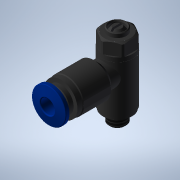
# Autodesk Inventor part: 193138 GRLA-M5-QS-4-D
Saved by Autodesk Inventor 2021 (Build 250183000, 183)
## iProperties
Created: 2026-04-07
Part Number: 193138 GRLA-M5-QS-4-D
Material: Generic
Catalog Web Link: www.3dfindit.com
Description: GRLA-D-one-way flow control valve
Vendor: FESTO
Document SubType Name: Modeling
Designer: psAdmin
Manufacturer: FESTO
Mass: 13 g
Surface Area: 17.273 cm^2
Volume: 2.07274 cm^3
Density: 1 g/cm^3
Appearance: PSOLRGB-176-176-176
Category: PARTsolutions
Company: FESTO
Title: 193138 GRLA-M5-QS-4-D
Author: Cadenas PARTsolutions
Comments: one-way flow control valve
PSOL_IDENT_0: {$CADENAS_DATA/23d-libs/festo/parts/g/grla/grla_d.prj},182 {VTYP=3D},{NB=193138 GRLA-M5-QS-4-D},{LIN
PSOL_IDENT_1: A=193138 GRLA-M5-QS-4-D},{NN=GRLA-D},{DATE=02.05.2025 09:35:38},{GEOMDATE=20.03.2025 09:32:41},{VERS
PSOL_IDENT_2: ION=},{LINEID=20},{WBVAR=},{WBNUMERIC=}  {NB=193138 GRLA-M5-QS-4-D},{LINA=193138 GRLA-M5-QS-4-D},{KT=
PSOL_IDENT_3: DUMMY},{TNR=193138},{TYP=GRLA-M5-QS-4-D},{INFO=},{FDTQS=46},{FDTQSV2=46},{FDTQS1=34},{FDTQS2=346},{F
PSOL_IDENT_4: DTQSDGST=-},{ZOLL=5},{VERS=1.000},{D=M5},{QS=QS-4},{ESTE=-},{DFC=-},{B=9.800},{DP=5.000},{KDRD=4.018
PSOL_IDENT_5: },{D1=8.900},{D2=10.000},{DS=4.000},{H=24.700},{H1=20.300},{L=20.800},{L1=3.350},{L2=10.700},{SW=8.0
PSOL_IDENT_6: 00},{CNSMASSEXACT=0.01300},{MOM=0.8 ±0.1},{GB=0.500},{LHT=1.200},{TW=0.700},{DW=8.400},{DHT=5.200},{
PSOL_IDENT_7: DCH=7.500},{DH=8.900},{HH=4.750},{HHB=5.950},{DI=2.000},{DIH=4.200},{LIH=0.400},{LTS=1.200},{DSJ1=7.
PSOL_IDENT_8: 200},{DSJ2=0.000},{TSJ=0.000},{LSJ1=5.450},{LSJ2=16.400},{ASJ=45.000},{LSJ3=1.815},{LSJ4=9.800},{LSJ
PSOL_IDENT_9: 5=3.300},{LSJ6=0.200},{DSJ3=4.200},{DSJ4=9.900},{DQS=0.000},{LQS=0.000},{DSJ5=7.500},{RSJ1=0.200},{R
PSOL_IDENT_10: SJ2=0.300},{DSJ6=5.400},{DSR=7.800},{TSR=0.500},{DSJ7=9.700},{HN=0.000},{DN=0.000},{DIN=0.000},{DNC=
PSOL_IDENT_11: 0.000},{CHN=0.000},{RN=0.000},{HKH=0.000},{DKH=0.000},{DIKH=0.000},{DKHC=0.000},{CHKH=0.000},{CHKH1=
PSOL_IDENT_12: 0.000},{RKH=0.000},{TKHS=0.000},{HSJ=0.000},{HSJN=0.000},{DAS=0.000},{TIH=1.520},{SRGH=0.150},{DISR=
PSOL_IDENT_13: 7.300},{TQS=15.000},{EOLDATE=},{GTIN=4052568043803},{REACH=Ja},{REACHSVHC=Nein},{REACHHAZSUBS=-},{RE
PSOL_IDENT_14: ACHSCIP=-},{REACHVALDATE=-}
NB: 193138 GRLA-M5-QS-4-D
NN: GRLA-D
NT: one-way flow control valve
NBSYN: $TNR. $TYP.
LINA: 193138 GRLA-M5-QS-4-D
CATALOG: Festo
TNR: 193138
TYP: GRLA-M5-QS-4-D
D: M5
QS: QS-4
ESTE: -
DFC: -
B: 9.8
D1: 8.9
D2: 10
DS: 4
H: 24.7
H1: 20.3
L: 20.8
L1: 3.35
L2: 10.7
SW: 8
CNSMASSEXACT: 0.013
MOM: 0.8 ±0.1
GTIN: 4052568043803
REACH: Yes
REACHSVHC: No
REACHHAZSUBS: -
REACHSCIP: -
REACHVALDATE: -
SUPPLIER: FESTO
ARTICLENO: 193138 GRLA-M5-QS-4-D
BOMINFO: 193138 GRLA-M5-QS-4-D
CREATOR: CADENAS GmbH
Autodesk Inventor part; units mm, degrees
sketch "Sketch_6" plane through (0, 0, 0) normal (0, 0, 1) x (1, 0, 0)
  line L0 (0, -14.05) -> (0, 10.1)
  line L1 (0, 10.1) -> (1.2, 10.1)
  line L2 (1.2, 10.1) -> (2.1, 8.9)
  line L3 (2.1, 8.9) -> (2.1, 9.7)
  line L4 (2.1, 9.7) -> (2.2865, 10.1)
  line L5 (2.2865, 10.1) -> (2.4, 10.1)
  line L6 (2.4, 10.1) -> (2.6, 9.9)
  line L7 (2.6, 9.9) -> (2.6, 8.9)
  line L8 (2.6, 8.9) -> (3.75, 8.9)
  line L9 (3.75, 8.9) -> (4.45, 8.4959)
  line L10 (4.45, 8.4959) -> (4.45, 4.15)
  line L11 (4.45, 4.15) -> (3.75, 4.15)
  line L12 (3.75, 4.15) -> (3.75, 4.1)
  line L13 (3.75, 4.1) -> (4.45, 4.1)
  line L14 (4.45, 4.1) -> (4.45, -9.65)
  line L15 (4.45, -9.65) -> (3.7264, -9.65)
  arc A0 (3.7264, -9.65) -> (3.95, -9.75) centre (3.95, -9.45) ccw
  line L16 (3.95, -9.75) -> (4.2, -9.75)
  line L17 (4.2, -9.75) -> (4.2, -10.45)
  line L18 (4.2, -10.45) -> (3.9, -10.45)
  line L19 (3.9, -10.45) -> (3.9, -10.7)
  line L20 (3.9, -10.7) -> (2.5, -10.7)
  line L21 (2.5, -10.7) -> (2.5, -13.5595)
  line L22 (2.5, -13.5595) -> (2.0095, -14.05)
  line L23 (2.0095, -14.05) -> (0, -14.05)
  line L24 (0, -14.05) -> (0, 10.1)
  constraints: 50 end point, 2 point on circle, 1 centre point
revolve "Revolution1" add sketch "Sketch_6" angle 360 about axis through (0, -14.05, 0) along (0, -1, 0)
thread "Thread1" size "M5x0.8" class "6g" standard "ISO Metric profile" full length
sketch "Sketch_8" plane through (0, 10.1, 0) normal (0, 1, 0) x (1, 0, 0)
  line L0 (-0.3, 1.9774) -> (-0.3, -1.9774)
  arc A0 (-0.3, -1.9774) -> (0.3, -1.9774) centre (0, 0) ccw
  line L1 (0.3, -1.9774) -> (0.3, 1.9774)
  arc A1 (0.3, 1.9774) -> (-0.3, 1.9774) centre (0, 0) ccw
  constraints: 4 end point, 4 point on circle, 2 centre point
extrude "Extrusion1" cut sketch "Sketch_8" against normal blind 1
sketch "Sketch_15" plane through (0, 10.1, 0) normal (0, 1, 0) x (1, 0, 0)
  line L0 (-8, -4.6188) -> (0, -9.2376)
  line L1 (0, -9.2376) -> (8, -4.6188)
  line L2 (8, -4.6188) -> (8, 4.6188)
  line L3 (8, 4.6188) -> (0, 9.2376)
  line L4 (0, 9.2376) -> (-8, 4.6188)
  line L5 (-8, 4.6188) -> (-8, -4.6188)
  line L6 (-4, -2.3094) -> (0, -4.6188)
  line L7 (0, -4.6188) -> (4, -2.3094)
  line L8 (4, -2.3094) -> (4, 2.3094)
  line L9 (4, 2.3094) -> (0, 4.6188)
  line L10 (0, 4.6188) -> (-4, 2.3094)
  line L11 (-4, 2.3094) -> (-4, -2.3094)
  constraints: 24 end point
extrude "Extrusion2" cut sketch "Sketch_15" against normal blind 4.75
sketch "Sketch_11" plane through (0, 0, 0) normal (1, 0, 0) x (0, 1, 0)
  line L0 (0, 0) -> (0, 20.3)
  line L1 (0, 20.3) -> (2.3, 20.3)
  line L2 (2.3, 20.3) -> (4.7847, 19.8619)
  arc A0 (4.95, 19.6649) -> (4.7847, 19.8619) centre (4.75, 19.6649) ccw
  line L3 (4.95, 19.6649) -> (4.95, 18.8)
  line L4 (4.95, 18.8) -> (3.1, 18.8)
  arc A1 (3.1, 18.8) -> (2.7, 18.4) centre (3.1, 18.4) ccw
  line L5 (2.7, 18.4) -> (2.7, 17.8)
  line L6 (2.7, 17.8) -> (3.55, 17.8)
  line L7 (3.55, 17.8) -> (3.75, 17.6)
  line L8 (3.75, 17.6) -> (3.75, 16.4)
  line L9 (3.75, 16.4) -> (4.85, 16.4)
  line L10 (4.85, 16.4) -> (4.85, 14.9)
  line L11 (4.85, 14.9) -> (5, 14.6402)
  line L12 (5, 14.6402) -> (5, 6.85)
  line L13 (5, 6.85) -> (3.6, 5.45)
  line L14 (3.6, 5.45) -> (3.6, 0)
  line L15 (3.6, 0) -> (0, 0)
  line L16 (0, 0) -> (0, 20.3)
  constraints: 34 end point, 4 point on circle, 2 centre point
revolve "Revolution2" add sketch "Sketch_11" angle 360 about axis through (0, 0, 0) along (0, 0, -1)
sketch "Sketch_10" plane through (0, 0, 0) normal (0, 0, 1) x (1, 0, 0)
  line L0 (-9.8, 34.2) -> (-9.8, -25.8)
  line L1 (-9.8, -25.8) -> (9.8, -25.8)
  line L2 (9.8, -25.8) -> (9.8, 34.2)
  line L3 (9.8, 34.2) -> (-9.8, 34.2)
  line L4 (-4.9, 29.2) -> (-4.9, -20.8)
  line L5 (-4.9, -20.8) -> (4.9, -20.8)
  line L6 (4.9, -20.8) -> (4.9, 29.2)
  line L7 (4.9, 29.2) -> (-4.9, 29.2)
  constraints: 16 end point
extrude "Extrusion3" cut sketch "Sketch_10" along normal blind 18.3
sketch "Sketch_5" plane through (0, 0, 0) normal (1, 0, 0) x (0, 1, 0)
  line L0 (0, 0) -> (0, 20.3)
  line L1 (0, 20.3) -> (2.3, 20.3)
  arc A0 (2.3, 20.3) -> (2, 20) centre (2.3, 20) ccw
  line L2 (2, 20) -> (2, 5.3)
  line L3 (2, 5.3) -> (1, 5.3)
  line L4 (1, 5.3) -> (1, 0)
  line L5 (1, 0) -> (0, 0)
  line L6 (0, 0) -> (0, 20.3)
  constraints: 14 end point, 2 point on circle, 1 centre point
revolve "Revolution3" cut sketch "Sketch_5" angle 360 about axis through (0, 0, 0) along (0, 0, -1)
sketch "Sketch7" plane through (0, -14.05, 0) normal (0, -1, 0) x (1, 0, 0)
  point P0 (0, 0)
hole "Hole1" at (0, -14.05, 0) direction (0, 1, 0) diameter 2 depth 16.05 countersink diameter 2.3464 countersink angle 60
ref_plane "FDT_MOUNT_XY" through (0, -10.7, 0) normal (0, 1, 0) x (-1, 0, 0)
ref_plane "FDT_MOUNT_YZ" through (0, -10.7, 0) normal (-1, 0, 0) x (0, 0, 1)
ref_plane "FDT_MOUNT_ZX" through (0, -10.7, 0) normal (0, 0, 1) x (0, 1, 0)
ref_plane "FDT_SCHLAUCH_XY" through (0, 0, 5.3) normal (0, 0, 1) x (1, 0, 0)
ref_plane "FDT_SCHLAUCH_YZ" through (0, 0, 5.3) normal (1, 0, 0) x (0, 1, 0)
ref_plane "FDT_SCHLAUCH_ZX" through (0, 0, 5.3) normal (0, 1, 0) x (0, 0, 1)
ref_plane "Zylinder_XY" through (0, -14.05, 0) normal (0, 1, 0) x (1, 0, 0)
ref_plane "Zylinder_YZ" through (0, -14.05, 0) normal (1, 0, 0) x (0, 0, -1)
ref_plane "Zylinder_ZX" through (0, -14.05, 0) normal (0, 0, -1) x (0, 1, 0)
ref_plane "anbau_XY" through (0, -10.7, 0) normal (0, 1, 0) x (1, 0, 0)
ref_plane "anbau_YZ" through (0, -10.7, 0) normal (1, 0, 0) x (0, 0, -1)
ref_plane "anbau_ZX" through (0, -10.7, 0) normal (0, 0, -1) x (0, 1, 0)
body "Solid1"
